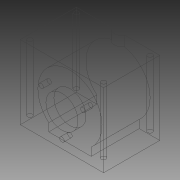
# Autodesk Inventor part: EncoderSupportInside
Saved by Autodesk Inventor 2014 SP1 (Build 180222100, 222)
## iProperties
Created: 2015-03-28
Part Number: EncoderSupportInside
Material: Generic
Document SubType Name: Modeling
Designer: david
Density: 1 g/cm^3
Appearance: Default
EncoderSupportInside_Length: 35,000 mm
EncoderSupportInside_Width: 52,000 mm
EncoderSupportInside_Height: 46,000 mm
EncoderSupportInside_Thickness: 6,000 mm
EncoderSupport_FixationHole_Diameter: 3,000 mm
EncoderSupport_FixationHole_Margin: 3,000 mm
Author: david
Autodesk Inventor part; units mm, degrees
ref_plane "YZ Plane" through (0, 0, 0) normal (1, 0, 0) x (0, 1, 0)
ref_plane "XZ Plane" through (0, 0, 0) normal (0, 1, 0) x (-1, 0, 0)
ref_plane "XY Plane" through (0, 0, 0) normal (0, 0, 1) x (1, 0, 0)
sketch "FrontSketch" plane through (0, 0, 0) normal (0, 0, 1) x (1, 0, 0)
  line L0 (0, 0) -> (0, 22.8261) construction
  line L1 (0, 0) -> (24.783, 0) construction
  circle A0 centre (0, 0) radius 10
  circle A1 centre (0, 0) radius 20 construction
  line L2 (-26, 26) -> (26, 26)
  line L3 (26, 26) -> (26, -20)
  line L4 (26, -20) -> (-26, -20)
  line L5 (-26, -20) -> (-26, 26)
  line L6 (0, 0) -> (-39.7334, 0) construction
  circle A2 centre (0, 0) radius 15 construction
  circle A3 centre (0, -15) radius 1.4
  line L7 (0, 0) -> (0, -25.6264) construction
  circle A4 centre (12.9904, 7.5) radius 1.4
  circle A5 centre (-12.9904, 7.5) radius 1.4
  point P0 (0, 20)
  point P1 (-20, 0)
  dimension "d25" = 30
  dimension "d21" = 20
  dimension "d22" = 40
  dimension "d23" = 6
  dimension "d24" = 6
  dimension "d26" = 2.8
  dimension "d29" = 360
  constraints: 16 end point, 5 centre point, 5 coincident, 4 perpendicular, 3 point on line, 2 parallel, 2 point on circle, 1 horizontal, 1 tangent, 1 vertical alignment, 10 other
  measures "d21" diameter of A0
  measures "d22" diameter of A1
  measures "d23" distance from line of L5 A1.start
  measures "d24" distance from line of L2 A1.end
  measures "d26" diameter of A3
extrude "Front" add sketch "FrontSketch" along normal blind 5
sketch "FerruleSketch" plane through (0, 0, 0) normal (0, 0, -1) x (-1, 0, 0)
  circle A0 centre (0, 0) radius 10 projected
  line L0 (26, 26) -> (-26, 26) projected
  line L1 (-26, 26) -> (-26, -20) projected
  line L2 (-26, -20) -> (26, -20) projected
  line L3 (26, -20) -> (26, 26) projected
  circle A1 centre (0, 0) radius 20
  dimension "d33" = 40
  constraints: 1 centre point, 1 coincident
  measures "d33" diameter of A1
extrude "Ferrule" add sketch "FerruleSketch" along normal blind 30 contours L3 L2 L1 L0
sketch "Sketch7" plane through (0, 0, -30) normal (0, 0, -1) x (-1, 0, 0)
  line L0 (-26, -20) -> (26, -20) projected
  circle A0 centre (0, 0) radius 20 projected
  line L1 (-26, -20) -> (26, -20) projected
  line L2 (26, -20) -> (26, 26) projected
  line L3 (13.2288, -15) -> (13.2288, -20)
  line L4 (-13.2288, -15) -> (-13.2288, -20)
  line L5 (0, 0) -> (0, -25.3199) construction
  point P0 (0, -20)
  dimension "d37" = 5
  constraints: 6 end point, 3 parallel, 2 point on circle, 2 point on line, 1 other
  measures "d37" distance of L3.start L3.end
extrude "Extrusion8" cut sketch "Sketch7" against normal up to surface (30 mm away) contours L4 A0 L0 | A0 L3 L0
sketch "CableHoleSketch" plane through (-26, 26, 5) normal (0, 1, 0) x (1, 0, 0)
  line L0 (0, 35) -> (52, 35) projected
  line L1 (26, 5) -> (26, 36.9321) construction
  circle A0 centre (26, 37) radius 4.5
  line L2 (46, 5) -> (6, 5) projected
  line L3 (21.9689, 35) -> (30.0311, 35)
  point P0 (12.7712, 5)
  point P1 (39.2288, 5)
  dimension "d40" = 32
  dimension "d41" = 9
  constraints: 4 end point, 3 point on line, 2 point on circle, 1 centre point, 1 perpendicular
  measures "d40" distance from line of L2 A0.centre
  measures "d41" diameter of A0
extrude "CableHole" cut sketch "CableHoleSketch" against normal up to next contours L0 A0 picked at (25.8154, 34.1781)
sketch "FixationHoleSketch" plane through (-26, 26, 5) normal (0, 1, 0) x (1, 0, 0)
  arc A0 (21.9689, 35) -> (30.0311, 35) centre (26, 37) ccw projected
  line L0 (30.0311, 35) -> (52, 35) projected
  circle A1 centre (3, 3) radius 1.5
  line L1 (26, 5) -> (26, 37) construction
  line L2 (52, 0) -> (0, 0) projected
  line L3 (52, 0) -> (52, 35) projected
  line L4 (-10.6096, 17.5) -> (55.9901, 17.5) construction
  circle A2 centre (3, 32) radius 1.5
  line L5 (26, 30) -> (26, -2) construction
  circle A3 centre (49, 3) radius 1.5
  circle A4 centre (49, 32) radius 1.5
  dimension "d44" = 3
  dimension "d45" = 3
  dimension "d52" = 23
  dimension "d53" = 17.5
  constraints: 6 end point, 5 symmetric about line, 4 centre point, 2 perpendicular, 3 other
  measures "d44" diameter of A1
  measures "d45" horizontal distance of L2.end A1.centre
  measures "d52" distance from line of L1 A1.centre
  measures "d53" distance between parallel lines of L2 L4
extrude "FixationHole" cut sketch "FixationHoleSketch" against normal blind 41
equation "\"d25\" = 2 * Encoder_FixationHole_DistanceToCenter"
equation "\"d21\" = Encoder_Bearing_Diameter"
equation "\"d22\" = Encoder_Body_Diameter"
equation "\"d23\" = EncoderSupportInside_Thickness"
equation "\"d24\" = EncoderSupportInside_Thickness"
equation "\"d26\" = Encoder_FixationHole_Size"
equation "\"d31\" = Encoder_Bearing_Height"
equation "\"d33\" = Encoder_Body_Diameter"
equation "\"d40\" = Encoder_CableFixation_DistanceToTop"
equation "\"d41\" = Encoder_CableFixation_Diameter"
equation "\"d44\" = EncoderSupport_FixationHole_Diameter"
equation "\"d45\" = EncoderSupport_FixationHole_Margin"
equation "\"d52\" = 0.5 * EncoderSupportInside_Width - EncoderSupport_FixationHole_Margin"
equation "\"d53\" = 0.5 * EncoderSupportInside_Length"
equation "\"EncoderSupportInside_Thickness\" = 6"
equation "\"EncoderSupportInside_Length\" = d31 + d34"
equation "\"EncoderSupportInside_Width\" = Encoder_Body_Diameter + 2 * EncoderSupportInside_Thickness"
equation "\"EncoderSupportInside_Height\" = Encoder_Body_Diameter + EncoderSupportInside_Thickness"
equation "\"EncoderSupport_FixationHole_Diameter\" = 3"
equation "\"EncoderSupport_FixationHole_Margin\" = 3"
equation "\"Encoder_FixationHole_DistanceToCenter\" = 15"
equation "\"Encoder_Bearing_Diameter\" = 20"
equation "\"Encoder_Body_Diameter\" = 40"
equation "\"Encoder_FixationHole_Size\" = 2.8"
equation "\"Encoder_Bearing_Height\" = 5"
equation "\"Encoder_CableFixation_DistanceToTop\" = 32"
equation "\"Encoder_CableFixation_Diameter\" = 9"
equation "\"d34\" = 30"
body "Solid2"
